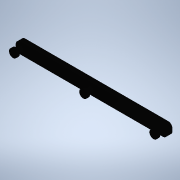
# Autodesk Inventor part: Lenkung_hinten_verbindung
Saved by Autodesk Inventor 2020 (Build 240168000, 168)
## iProperties
Created: 2020-02-20
Part Number: Lenkung_hinten_verbindung
Material: Generisch
Document SubType Name: Modeling
Designer: Stefan
Density: 1 g/cm^3
Appearance: Vorgabe
Mass: 60.4772 g
Surface Area: 192.13 cm^2
Volume: 60.4772 cm^3
Author: Stefan
Autodesk Inventor part; units mm, degrees
ref_plane "YZ Plane" through (0, 0, 0) normal (1, 0, 0) x (0, 1, 0)
ref_plane "XZ Plane" through (0, 0, 0) normal (0, 1, 0) x (-1, 0, 0)
ref_plane "XY Plane" through (0, 0, 0) normal (0, 0, 1) x (1, 0, 0)
sketch "Skizze1" plane through (0, 0, 0) normal (0, 0, 1) x (1, 0, 0)
  circle A0 centre (0, 0) radius 4.95
  circle A1 centre (-130, 0) radius 4.95
  circle A2 centre (130, 0) radius 4.95
  dimension "d0" = 9.9
  dimension "d1" = 9.9
  dimension "d2" = 130
  dimension "d3" = 9.9
  dimension "d4" = 130
  constraints: 3 centre point, 1 coincident
  measures "d0" diameter of A0
  measures "d1" diameter of A1
  measures "d2" distance of point (0, 0) A1.centre
  measures "d3" diameter of A2
  measures "d4" distance of A2.centre point (0, 0)
extrude "Extrusion1" add sketch "Skizze1" along normal blind 10
sketch "Skizze2" plane through (0, 0, 0) normal (0, 0, -1) x (-1, 0, 0)
  line L0 (132.5, -10) -> (-132.5, -10)
  line L1 (-140, -2.5) -> (-140, 2.5)
  line L2 (-132.5, 10) -> (132.5, 10)
  line L3 (140, 2.5) -> (140, -2.5)
  arc A0 (132.5, -10) -> (140, -2.5) centre (132.5, -2.5) ccw
  arc A1 (140, 2.5) -> (132.5, 10) centre (132.5, 2.5) ccw
  arc A2 (-132.5, 10) -> (-140, 2.5) centre (-132.5, 2.5) ccw
  arc A3 (-140, -2.5) -> (-132.5, -10) centre (-132.5, -2.5) ccw
  point P0 (0, 0)
  point P1 (140, -10)
  point P2 (-140, -10)
  point P3 (140, 10)
  dimension "d7" = 20
  dimension "d8" = 280
  dimension "d9" = 140
  dimension "d10" = 7.5
  dimension "d11" = 10
  constraints: 8 end point, 8 point on circle, 8 tangent, 6 point on line, 4 centre point, 3 equal radius, 2 parallel, 1 horizontal, 1 perpendicular
  measures "d7" distance of point (140, 10) point (140, -10)
  measures "d8" distance of point (140, -10) point (-140, -10)
  measures "d9" horizontal distance of point (0, 0) point (-140, -10)
  measures "d10" radius of A0
  measures "d11" vertical distance of point (0, 0) point (140, -10)
extrude "Extrusion2" add sketch "Skizze2" along normal blind 10
sketch "Skizze3" plane through (0, 0, 10) normal (0, 0, 1) x (1, 0, 0)
  circle A0 centre (0, 0) radius 7.5
  circle A1 centre (130, 0) radius 7.5
  circle A2 centre (-130, 0) radius 4.95 projected
  circle A3 centre (-130, 0) radius 7.5
  dimension "d14" = 15
  dimension "d15" = 15
  dimension "d16" = 130
  dimension "d17" = 0
  dimension "d18" = 15
  constraints: 3 centre point, 2 coincident
  measures "d14" diameter of A0
  measures "d15" diameter of A1
  measures "d16" distance of point (0, 0) A1.centre
  measures "d17" vertical distance of point (0, 0) A1.centre
  measures "d18" diameter of A3
extrude "Extrusion3" add sketch "Skizze3" along normal blind 5 contours A0 | A1 | A2 | A3
